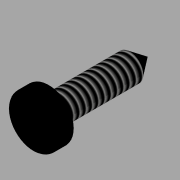
# Autodesk Inventor part: M1.7_6mm self-tapping screw
Saved by Autodesk Inventor 2019 (Build 230136000, 136)
## iProperties
Created: 2019-02-12
Part Number: M1.7_6mm self-tapping screw
Material: Generic
Document SubType Name: Modeling
Designer: Ben
Density: 1 g/cm^3
Appearance: Default
Author: Ben
Autodesk Inventor part; units mm, degrees
ref_plane "YZ Plane" through (0, 0, 0) normal (1, 0, 0) x (0, 1, 0)
ref_plane "XZ Plane" through (0, 0, 0) normal (0, 1, 0) x (-1, 0, 0)
ref_plane "XY Plane" through (0, 0, 0) normal (0, 0, 1) x (1, 0, 0)
sketch "Sketch1" plane through (0, 0, 0) normal (0, 0, 1) x (1, 0, 0)
  circle A0 centre (0, 0) radius 0.75
  dimension "d0" = 1.5
  constraints: 1 centre point, 1 coincident
  measures "d0" diameter of A0
extrude "Extrusion1" add sketch "Sketch1" against normal blind 5.5
sketch "Sketch2" plane through (0, 0, 0) normal (0, 0, 1) x (1, 0, 0)
  circle A0 centre (0, 0) radius 1.425
  dimension "d3" = 2.85
  constraints: 1 centre point, 1 coincident
  measures "d3" diameter of A0
extrude "Extrusion2" add sketch "Sketch2" along normal blind 0.95
chamfer "Chamfer1" distance 0.75 distance2 1 1 edges at (-0.75, 0, -5.5) measured on face at (0.5185, -0.1278, -5.5)
fillet "Fillet1" radius 0.2 1 edges at (-1.425, 0, 0.95)
fillet "Fillet2" radius 0.1 1 edges at (-1.425, 0, 0)
sketch "Sketch3" plane through (0, 0, 0.95) normal (0, 0, 1) x (1, 0, 0)
  line L0 (1.25, 0.125) -> (-1.25, 0.125)
  line L1 (-1.25, 0.125) -> (-1.25, -0.125)
  line L2 (-1.25, -0.125) -> (1.25, -0.125)
  line L3 (1.25, -0.125) -> (1.25, 0.125)
  line L4 (1.25, 0.125) -> (-1.25, -0.125) construction
  line L5 (-1.25, 0.125) -> (1.25, -0.125) construction
  line L6 (0.125, -1.25) -> (-0.125, -1.25)
  line L7 (-0.125, -1.25) -> (-0.125, 1.25)
  line L8 (-0.125, 1.25) -> (0.125, 1.25)
  line L9 (0.125, 1.25) -> (0.125, -1.25)
  line L10 (0.125, -1.25) -> (-0.125, 1.25) construction
  line L11 (-0.125, -1.25) -> (0.125, 1.25) construction
  point P0 (0, 0)
  point P1 (0, 0)
  dimension "d11" = 2.5
  dimension "d12" = 0.25
  dimension "d13" = 0.25
  dimension "d14" = 2.5
  constraints: 24 end point, 4 midpoint, 4 parallel, 2 horizontal, 2 perpendicular
  measures "d11" distance of L2.end L1.end
  measures "d12" distance of L1.end L0.end
  measures "d13" distance of L7.end L8.end
  measures "d14" distance of L6.end L7.end
extrude "Extrusion3" cut sketch "Sketch3" against normal blind 0.25
thread "Thread1" size "M1.7x0.35" class "6g" standard "ANSI Metric M Profile" full length
equation "\"d6\" = 0.5 * d0"
body "Solid1"
